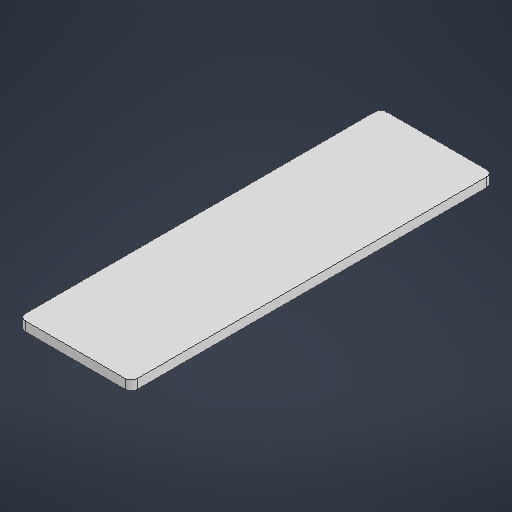
# Autodesk Inventor part: module-lid_switch
Saved by Autodesk Inventor 2025.2 (Build 292293000, 293)
## iProperties
Created: 2025-09-07
Part Number: module-lid_switch
Material: Generic
Document SubType Name: Modeling
Designer: sam
Density: 1 g/cm^3
Appearance: Default
Author: sam
Autodesk Inventor part; units mm, degrees
ref_plane "YZ Plane" through (0, 0, 0) normal (1, 0, 0) x (0, 1, 0)
ref_plane "XZ Plane" through (0, 0, 0) normal (0, 1, 0) x (-1, 0, 0)
ref_plane "XY Plane" through (0, 0, 0) normal (0, 0, 1) x (1, 0, 0)
sketch "Sketch1" plane through (0, 0, 0) normal (0, 1, 0) x (-1, 0, 0)
  line L0 (-18, -58) -> (18, -58)
  line L1 (18, -58) -> (18, 58)
  line L2 (18, 58) -> (-18, 58)
  line L3 (-18, 58) -> (-18, -58)
  line L4 (-18, -58) -> (18, 58) construction
  line L5 (18, -58) -> (-18, 58) construction
  point P0 (0, 0)
  dimension "d0" = 36
  dimension "d1" = 116
  constraints: 12 end point, 2 midpoint, 2 parallel, 1 horizontal, 1 perpendicular
  measures "d0" distance of L2.end L1.end
  measures "d1" distance between parallel lines of L0 L2
extrude "Extrusion1" add sketch "Sketch1" along normal blind 3
sketch "Sketch2" plane through (0, 0, 0) normal (0, -1, 0) x (1, 0, 0)
  line L0 (15, 55) -> (-15, 55)
  line L1 (-15, 55) -> (-15, -55)
  line L2 (-15, -55) -> (15, -55)
  line L3 (15, -55) -> (15, 55)
  line L4 (15, 55) -> (-15, -55) construction
  line L5 (-15, 55) -> (15, -55) construction
  line L6 (-18, -58) -> (-18, 58) projected
  line L7 (18, -58) -> (-18, -58) projected
  point P0 (0, 0)
  dimension "d4" = 3
  dimension "d5" = 3
  constraints: 12 end point, 2 midpoint, 2 parallel, 1 horizontal, 1 perpendicular
  measures "d4" distance between parallel lines of L6 L1
  measures "d5" distance between parallel lines of L7 L2
extrude "Extrusion2" add sketch "Sketch2" along normal blind 3
fillet "Fillet1" radius 2 8 edges at (18, 1.5, 58) (15, -1.5, 55) (-15, -1.5, 55) (-18, 1.5, 58) (15, -1.5, -55) (18, 1.5, -58) (-18, 1.5, -58) (-15, -1.5, -55)
body "Solid1"
